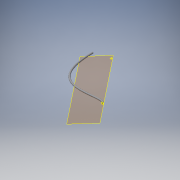
# Autodesk Inventor part: Pi Wire
Saved by Autodesk Inventor 2018 (Build 220112000, 112)
## iProperties
Created: 2018-07-20
Part Number: Pi Wire
Material: Generic
Document SubType Name: Modeling
Designer: DPLXuser
Density: 1 g/cm^3
Appearance: Default
Author: DPLXuser
Autodesk Inventor part; units mm, degrees
ref_plane "YZ Plane" through (0, 0, 0) normal (1, 0, 0) x (0, 1, 0)
ref_plane "XZ Plane" through (0, 0, 0) normal (0, 1, 0) x (-1, 0, 0)
ref_plane "XY Plane" through (0, 0, 0) normal (0, 0, 1) x (1, 0, 0)
ref_plane "Work Plane1" through (9.7636, 5.7071, -125.5411) normal (0, 0, -1) x (-1, 0, 0)
sketch "Sketch1" plane through (9.7636, 5.7071, -125.5411) normal (0, 0, -1) x (-1, 0, 0)
  circle A0 centre (0, 0) radius 2
  point P0 (9.7636, -5.7071)
  dimension "d0" = 4
  constraints: 1 centre point
  measures "d0" diameter of A0
ref_plane "Work Plane2" through (9.7636, 5.7071, -125.5411) normal (-0.1378, 0.9905, -0.0049) x (-0.6313, -0.0916, -0.7701)
sketch "Sketch2" plane through (9.7636, 5.7071, -125.5411) normal (-0.1378, 0.9905, -0.0049) x (-0.6313, -0.0916, -0.7701)
  line L0 (0, 0) -> (9.0069, -5.3655) construction
  line L1 (9.0069, -5.3655) -> (45.973, 47.2607) construction
  line L2 (45.973, 47.2607) -> (92.679, 95.1583) construction
  line L3 (92.679, 95.1583) -> (156.8325, 59.5525) construction
  line L4 (156.8325, 59.5525) -> (186.9093, 36.0208) construction
  spline S0 degree 4 poles (0, 0) (9.0069, -5.3655) (45.973, 47.2607) (92.679, 95.1583) (156.8325, 59.5525) (186.9093, 36.0208) knots 1 1 1 1 1 2 3 3 3 3 3
  point P0 (-89.9947, 88.1201)
  constraints: 3 other
sweep "Sweep1" add profiles "Sketch1" path "Sketch2"
body "Solid1"
